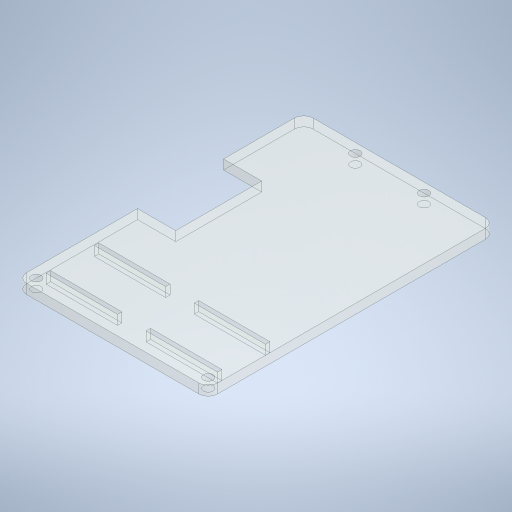
# Autodesk Inventor part: BaseS
Saved by Autodesk Inventor 2024 (Build 280153020, 153B)
## iProperties
Created: 2023-05-25
Part Number: BaseS
Material: Genérico
Document SubType Name: Modeling
Designer: victo
Density: 1 g/cm^3
Appearance: Transparente
Author: victo
Autodesk Inventor part; units mm, degrees
ref_plane "YZ Plane" through (0, 0, 0) normal (1, 0, 0) x (0, 1, 0)
ref_plane "XZ Plane" through (0, 0, 0) normal (0, 1, 0) x (-1, 0, 0)
ref_plane "XY Plane" through (0, 0, 0) normal (0, 0, 1) x (1, 0, 0)
sketch "Esboço1" plane through (0, 0, 0) normal (0, 1, 0) x (-1, 0, 0)
  line L0 (0, 0) -> (0, -150)
  line L1 (0, -150) -> (100, -150)
  line L2 (100, -150) -> (100, 0)
  line L3 (100, 0) -> (0, 0)
  dimension "d0" = 150
  dimension "d1" = 100
  constraints: 8 end point, 3 perpendicular, 1 vertical
  measures "d0" distance of L0.start L0.end
  measures "d1" distance of L0.end L1.end
extrude "Extrusão1" add sketch "Esboço1" along normal blind 5
fillet "Arredondamento1" radius 5 1 edges at (0, 2.5, 0)
fillet "Arredondamento2" radius 5 1 edges at (-100, 2.5, 0)
fillet "Arredondamento3" radius 5 2 edges at (-100, 2.5, -150) (0, 2.5, -150)
sketch "Esboço2" plane through (0, 5, 0) normal (0, 1, 0) x (1, 0, 0)
  circle A0 centre (-5, 5) radius 2.5
  circle A1 centre (-95, 5) radius 2.5
  circle A2 centre (-68, 145) radius 2.5
  circle A3 centre (-32, 145) radius 2.5
  circle A4 centre (-5, 5) radius 2.5
  dimension "d26" = 5
  dimension "d28" = 5
  dimension "d41" = 5
  dimension "d42" = 5
  constraints: 5 centre point, 2 coincident, 1 concentric
  measures "d26" diameter of A0
  measures "d28" diameter of A1
  measures "d41" diameter of A2
  measures "d42" diameter of A3
sketch "Esboço3" plane through (0, 5, 0) normal (0, 1, 0) x (1, 0, 0)
  line L0 (-5, 150) -> (-95, 150) projected
  line L1 (-80, 108) -> (-80, 63)
  line L2 (-100, 145) -> (-100, 5) projected
  line L3 (-80, 108) -> (-106.6116, 108)
  line L4 (-80, 63) -> (-106.6116, 63)
  circle A0 centre (-32, 145) radius 2.5 projected
  line L5 (-67.9453, 145) -> (-32, 145)
  point P0 (0, 0)
  point P1 (-100, 108)
  point P2 (-100, 63)
  point P3 (-100, 108)
  point P4 (-100, 63)
  dimension "d53" = 45
  constraints: 8 end point, 3 horizontal, 2 point on line, 1 vertical
  measures "d53" distance between parallel lines of L4 L3
extrude "Extrusão9" cut sketch "Esboço3" against normal through all contours L1 L4 L2 L3
extrude "Extrusão10" cut sketch "Esboço2" against normal through all
sketch "Esboço4" plane through (0, 5, 0) normal (0, 1, 0) x (1, 0, 0)
  line L0 (-95, 0) -> (-5, 0) projected
  line L1 (-5, 34.9997) -> (-42.3, 34.9997)
  line L2 (-42.3, 12.0997) -> (-5, 12.0997)
  line L3 (-42.3, 12.0997) -> (-42.3, 9.7997)
  line L4 (-42.3, 9.7997) -> (-5, 9.7997)
  line L5 (-5, 9.7997) -> (-5, 12.0997)
  line L6 (-5, 34.9997) -> (-5, 37.2997)
  line L7 (-5, 37.2997) -> (-42.3, 37.2997)
  line L8 (-42.3, 37.2997) -> (-42.3, 34.9997)
  line L9 (-57.3, 34.9997) -> (-94.6, 34.9997)
  line L10 (-94.6, 12.0997) -> (-57.3, 12.0997)
  line L11 (-94.6, 12.0997) -> (-94.6, 9.7997)
  line L12 (-94.6, 9.7997) -> (-57.3, 9.7997)
  line L13 (-57.3, 9.7997) -> (-57.3, 12.0997)
  line L14 (-57.3, 34.9997) -> (-57.3, 37.2997)
  line L15 (-57.3, 37.2997) -> (-94.6, 37.2997)
  line L16 (-94.6, 37.2997) -> (-94.6, 34.9997)
  point P0 (0, 0)
  dimension "d62" = 37.3
  dimension "d63" = 22.9
  dimension "d64" = 2.3
  dimension "d65" = 2.3
  dimension "d67" = 37.3
  constraints: 32 end point, 8 perpendicular, 5 point on line, 1 horizontal, 1 vertical
  measures "d62" distance of L1.start L1.end
  measures "d63" distance of L1.end L2.start
  measures "d64" distance of L2.start L3.end
  measures "d65" distance of L1.start L6.end
  measures "d67" distance of L9.start L9.end
extrude "Extrusão11" cut sketch "Esboço4" against normal through all
